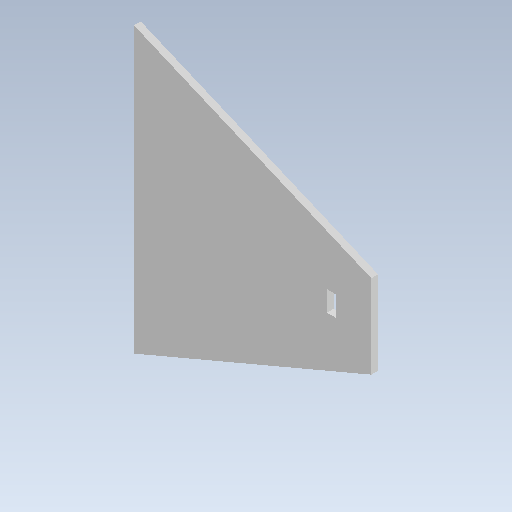
# Autodesk Inventor part: Pata
Saved by Autodesk Inventor 2020.1 (Build 241239000, 239)
## iProperties
Created: 2019-12-03
Part Number: Pata
Material: Generic
Document SubType Name: Modeling
Designer: Daniel
Density: 1 g/cm^3
Appearance: Default
Author: Daniel
Autodesk Inventor part; units mm, degrees
ref_plane "YZ Plane" through (0, 0, 0) normal (1, 0, 0) x (0, 1, 0)
ref_plane "XZ Plane" through (0, 0, 0) normal (0, 1, 0) x (-1, 0, 0)
ref_plane "XY Plane" through (0, 0, 0) normal (0, 0, 1) x (1, 0, 0)
sketch "Sketch1" plane through (0, 0, 0) normal (0, 0, 1) x (1, 0, 0)
  line L0 (20.6369, -45.2692) -> (20.6369, -8.7308) projected
  line L1 (0, 0) -> (20.6369, -8.7308) projected
  line L2 (0, -54) -> (0, 0) construction
  line L3 (20.6369, -8.7308) -> (-85, 35.9608)
  line L4 (0, -27) -> (20.6369, -27) construction
  line L5 (0, -54) -> (20.6369, -45.2692) projected
  line L6 (20.6369, -45.2692) -> (-85, -89.9608)
  line L7 (-85, 35.9608) -> (-85, -89.9608)
  line L8 (20.1369, -8.5193) -> (20.1369, -45.4807)
  line L9 (1, -31) -> (1, -23) projected
  line L10 (1, -31) -> (3.3419, -31) projected
  line L11 (3.3419, -23) -> (1, -23) projected
  line L12 (4.5, -31.5) -> (0.5, -31.5)
  line L13 (0.5, -31.5) -> (0.5, -22.5)
  line L14 (0.5, -22.5) -> (4.5, -22.5)
  line L15 (4.5, -22.5) -> (4.5, -31.5)
  line L16 (3.3419, -31) -> (3.3419, -23) projected
  dimension "d0" = 85
  dimension "d3" = 0.5
  dimension "d4" = 0.5
  constraints: 18 end point, 3 point on line, 2 midpoint, 1 symmetric about line, 1 vertical, 2 other
  measures "d0" distance between parallel lines of L7 L2
  measures "d3" distance between parallel lines of L0 L8
  measures "d4" distance between parallel lines of L10 L12
extrude "Extrusion1" add sketch "Sketch1" along normal blind 3 contours L5 L6 L7 L3 L1 L8
body "Solid1"
